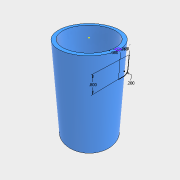
# Autodesk Inventor part: Adapter
Saved by Autodesk Inventor 2020.1 (Build 241239000, 239)
## iProperties
Created: 2019-10-18
Part Number: Adapter
Material: Aluminum 6061
Document SubType Name: Modeling
Designer: thom_tremblay
Density: 2.7 g/cm^3
Appearance: Cyan
Author: thom_tremblay
Autodesk Inventor part; units mm, degrees
ref_plane "XZ Plane" through (0, 0, 0) normal (0, 1, 0) x (-1, 0, 0)
ref_plane "XY Plane" through (0, 0, 0) normal (0, 0, 1) x (1, 0, 0)
sketch "Sketch1" plane through (0, 0, 0) normal (0, 1, 0) x (-1, 0, 0)
  circle A0 centre (0, 0) radius 38.1
  circle A1 centre (0, 0) radius 33.02
  dimension "d0" = 76.2
  dimension "d1" = 5.08
  constraints: 2 centre point, 1 coincident
  measures "d0" diameter of A0
  measures "d1" radial gap between concentric circles of A0 A1
extrude "Extrusion1" add sketch "Sketch1" against normal blind 127
ref_plane "Work Plane1" through (50.8, 0, 0) normal (1, 0, 0) x (0, 1, 0)
sketch "Sweep path" plane through (50.8, 0, 0) normal (1, 0, 0) x (0, 1, 0)
  line L0 (-20.32, 12.7) -> (-20.32, 5.08)
  arc A0 (-20.32, 5.08) -> (-15.24, 0) centre (-15.24, 5.08) ccw
  line L1 (-15.24, 0) -> (0, 0)
  dimension "d5" = 20.32
  dimension "d6" = 5.08
  dimension "d7" = 12.7
  constraints: 4 end point, 2 point on circle, 2 tangent, 1 centre point, 1 perpendicular, 1 vertical
  measures "d5" distance from line of L1.end L0
  measures "d6" radius of A0
  measures "d7" distance from line of L0.start L1
sketch "Sweep profile" plane through (0, 0, 0) normal (0, 1, 0) x (1, 0, 0)
  line L0 (34.6191, -1.2826) -> (38.6831, -1.2826)
  line L1 (38.6831, -1.2826) -> (38.6831, 4.0514)
  line L2 (38.6831, 4.0514) -> (34.6191, 4.0514)
  line L3 (34.6191, 4.0514) -> (34.6191, -1.2826)
  line L4 (34.6191, 1.3844) -> (38.6831, 1.3844) construction
  point P0 (0, 0)
  point P1 (36.6511, 1.3844)
  dimension "d8" = 2.032
  dimension "d9" = 5.334
  dimension "d11" = 5.08
  dimension "d12" = 38.1
  dimension "d13" = 58.42
  dimension "d14" = 17.78
  constraints: 8 end point, 8 point on circle, 8 tangent, 4 centre point, 3 equal radius, 2 parallel, 1 horizontal, 1 midpoint, 1 perpendicular, 1 vertical alignment
  measures "d12" distance from line of point (0, 0) L0
  measures "d13" distance between parallel lines of L2 L0
  measures "d14" distance between parallel lines of L3 L1
body "Solid1"
